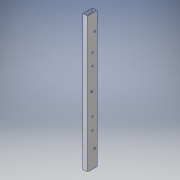
# Autodesk Inventor part: 1x2x28
Saved by Autodesk Inventor 2016 (Build 200138000, 138)
## iProperties
Created: 2016-01-16
Part Number: 1x2x28
Material: Aluminum 6061
Document SubType Name: Modeling
Designer: gus
Density: 2.7 g/cm^3
Appearance: Aluminum - Flat
Mass: 845.601 g
Surface Area: 1992.78 cm^2
Volume: 313.185 cm^3
Author: gus
Autodesk Inventor part; units mm, degrees
ref_plane "YZ Plane" through (0, 0, 0) normal (1, 0, 0) x (0, 1, 0)
ref_plane "XZ Plane" through (0, 0, 0) normal (0, 1, 0) x (-1, 0, 0)
ref_plane "XY Plane" through (0, 0, 0) normal (0, 0, 1) x (1, 0, 0)
sketch "Sketch1" plane through (0, 0, 0) normal (0, 1, 0) x (-1, 0, 0)
  line L0 (0, 0) -> (25.4, 0)
  line L1 (25.4, 0) -> (25.4, -50.8)
  line L2 (25.4, -50.8) -> (0, -50.8)
  line L3 (0, -50.8) -> (0, 0)
  line L4 (3.175, -3.175) -> (22.225, -3.175)
  line L5 (22.225, -3.175) -> (22.225, -47.625)
  line L6 (22.225, -47.625) -> (3.175, -47.625)
  line L7 (3.175, -47.625) -> (3.175, -3.175)
  dimension "d0" = 25.4
  dimension "d1" = 50.8
  dimension "d2" = 3.175
  constraints: 16 end point, 4 parallel, 2 perpendicular, 1 horizontal, 3 other
  measures "d0" distance of L1.end L2.end
  measures "d1" distance of L0.end L1.end
  measures "d2" distance between parallel lines of L3 L7
extrude "Extrusion1" add sketch "Sketch1" along normal blind 711.2
sketch "Sketch2" plane through (-25.4, 0, -50.8) normal (-1, 0, 0) x (0, 0, 1)
  circle A0 centre (28.575, 355.6) radius 4.7625
  line L0 (0, 711.2) -> (50.8, 711.2) projected
  line L1 (0, 0) -> (0, 711.2) projected
  circle A1 centre (12.7, 622.3) radius 4.7625
  line L2 (50.8, 0) -> (50.8, 711.2) projected
  circle A2 centre (12.7, 88.9) radius 4.7625
  line L3 (0, 88.9) -> (50.8, 88.9) construction
  line L4 (50.8, 0) -> (50.8, 711.2) projected
  line L5 (0, 622.3) -> (50.8, 622.3) construction
  circle A3 centre (25.4, 177.8) radius 3.3734
  line L6 (50.8, 0) -> (0, 0) projected
  circle A4 centre (25.4, 241.3) radius 3.3734
  circle A5 centre (25.4, 533.4) radius 3.3734
  circle A6 centre (25.4, 469.9) radius 3.3734
  dimension "d6" = 355.6
  dimension "d7" = 28.575
  dimension "d10" = 9.525
  dimension "d11" = 38.1
  dimension "d14" = 38.1
  dimension "d16" = 266.7
  dimension "d17" = 266.7
  dimension "d18" = 6.7469
  dimension "d19" = 25.4
  dimension "d20" = 177.8
  dimension "d22" = 241.3
  dimension "d23" = 25.4
  dimension "d25" = 25.4
  dimension "d26" = 177.8
  dimension "d28" = 25.4
  dimension "d29" = 241.3
  constraints: 7 centre point, 6 point on line, 5 equal radius, 4 end point, 1 horizontal, 1 perpendicular
  measures "d6" distance from line of A0.centre L0
  measures "d7" distance from line of L1 A0.centre
  measures "d10" diameter of A1
  measures "d11" distance from line of L2 A1.centre
  measures "d14" distance from line of L2 A2.centre
  measures "d16" distance from line of A0.centre L3
  measures "d17" distance from line of A0.centre L5
  measures "d18" diameter of A3
  measures "d19" distance from line of L1 A3.centre
  measures "d20" distance from line of L6 A3.centre
  measures "d22" distance from line of A4.centre L6
  measures "d23" distance from line of L1 A4.centre
  measures "d25" distance from line of L1 A5.centre
  measures "d26" distance from line of L0 A5.centre
  measures "d28" distance from line of L1 A6.centre
  measures "d29" distance from line of L0 A6.centre
extrude "Extrusion2" cut sketch "Sketch2" against normal blind 25.4 contours A0 | A1 | A2 | A3 | A4 | A5 | A6
sketch "Sketch3" plane through (0, 0, 0) normal (1, 0, 0) x (0, 0, -1)
  point P0 (0, 0)
body "Solid1"
